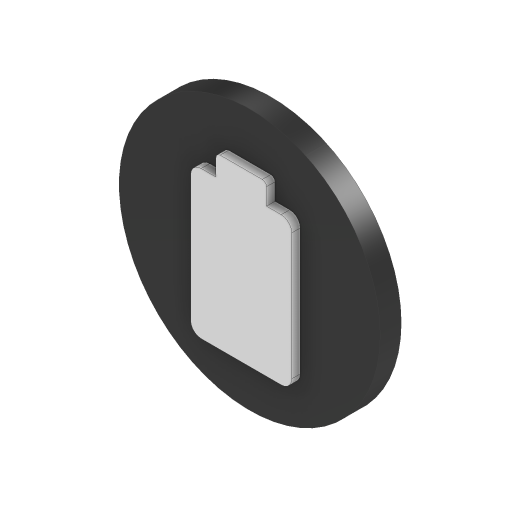
# Autodesk Inventor part: button_plate_battery
Saved by Autodesk Inventor 2023 (Build 270158000, 158)
## iProperties
Created: 2025-02-19
Part Number: button_plate_battery
Material: Všeobecné
Document SubType Name: Modeling
Designer: Marek
Density: 1 g/cm^3
Appearance: Výchozí
Author: Marek
Autodesk Inventor part; units mm, degrees
ref_plane "YZ Plane" through (0, 0, 0) normal (1, 0, 0) x (0, 1, 0)
ref_plane "XZ Plane" through (0, 0, 0) normal (0, 1, 0) x (-1, 0, 0)
ref_plane "XY Plane" through (0, 0, 0) normal (0, 0, 1) x (1, 0, 0)
sketch "Náčrt1" plane through (0, 0, 0) normal (0, 0, 1) x (1, 0, 0)
  line L0 (0, 8.68) -> (0, -8.68) projected
  line L1 (-8.68, 0) -> (8.68, 0) projected
  circle A0 centre (0, 0) radius 6.2
  dimension "d0" = 12.4
  constraints: 1 centre point, 1 coincident
  measures "d0" diameter of A0
extrude "Vysunutí1" add sketch "Náčrt1" along normal blind 1
sketch "Náčrt2" plane through (0, 0, 1) normal (0, 0, 1) x (1, 0, 0)
  line L0 (-8.68, 0) -> (8.68, 0) projected
  line L1 (0, 8.68) -> (0, -8.68) projected
  line L2 (-1.9, 3) -> (1.9, 3)
  line L3 (2.4, 2.5) -> (2.4, -3.5)
  line L4 (1.9, -4) -> (-1.9, -4)
  line L5 (-2.4, -3.5) -> (-2.4, 2.5)
  line L6 (-1.2, 3) -> (1.2, 3)
  line L7 (1.2, 3) -> (1.2, 3.8)
  line L8 (1, 4) -> (-1, 4)
  line L9 (-1.2, 3.8) -> (-1.2, 3)
  arc A0 (-1.9, 3) -> (-2.4, 2.5) centre (-1.9, 2.5) ccw
  arc A1 (2.4, 2.5) -> (1.9, 3) centre (1.9, 2.5) ccw
  arc A2 (-2.4, -3.5) -> (-1.9, -4) centre (-1.9, -3.5) ccw
  arc A3 (1.9, -4) -> (2.4, -3.5) centre (1.9, -3.5) ccw
  arc A4 (-1, 4) -> (-1.2, 3.8) centre (-1, 3.8) ccw
  arc A5 (1.2, 3.8) -> (1, 4) centre (1, 3.8) ccw
  point P0 (0, 0)
  dimension "d3" = 2.4
  dimension "d4" = 2.4
  dimension "d5" = 4
  dimension "d6" = 3
  dimension "d7" = 1.2
  dimension "d8" = 1.2
  dimension "d9" = 1
  dimension "d10" = 0.5
  dimension "d11" = 0.2
  constraints: 16 end point, 12 point on circle, 12 tangent, 6 centre point, 4 equal radius, 4 parallel, 2 horizontal, 2 perpendicular, 1 point on line
  measures "d3" distance between parallel lines of L1 L3
  measures "d4" distance between parallel lines of L5 L1
  measures "d5" distance between parallel lines of L0 L4
  measures "d6" distance between parallel lines of L2 L0
  measures "d7" distance between parallel lines of L1 L7
  measures "d8" distance between parallel lines of L9 L1
  measures "d9" distance between parallel lines of L2 L8
  measures "d10" radius of A0
  measures "d11" radius of A4
extrude "Vysunutí2" add sketch "Náčrt2" along normal blind 0.4
